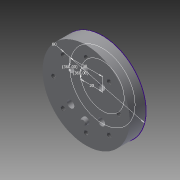
# Autodesk Inventor part: plate_for_CFS055CA501U
Saved by Autodesk Inventor 2013 (Build 170138000, 138)
## iProperties
Created: 2013-01-30
Part Number: plate_for_CFS055CA501U
Material: Generic
Document SubType Name: Modeling
Designer: Mahisorn
Density: 1 g/cm^3
Author: Mahisorn
Autodesk Inventor part; units mm, degrees
ref_plane "YZ Plane" through (0, 0, 0) normal (1, 0, 0) x (0, 1, 0)
ref_plane "XZ Plane" through (0, 0, 0) normal (0, 1, 0) x (-1, 0, 0)
ref_plane "XY Plane" through (0, 0, 0) normal (0, 0, 1) x (1, 0, 0)
sketch "Sketch1" plane through (0, 0, 0) normal (0, 1, 0) x (-1, 0, 0)
  circle A0 centre (0, 0) radius 40
  point P0 (20, 0)
  point P1 (14.1421, 14.1421)
  point P2 (0, 20)
  point P3 (-14.1421, 14.1421)
  point P4 (-20, 0)
  point P5 (-14.1421, -14.1421)
  point P6 (0, -20)
  point P7 (14.1421, -14.1421)
  point P8 (30, 0)
  point P9 (21.2132, 21.2132)
  point P10 (0, 30)
  point P11 (-21.2132, 21.2132)
  point P12 (-30, 0)
  point P13 (-21.2132, -21.2132)
  point P14 (0, -30)
  point P15 (21.2132, -21.2132)
  dimension "d0" = 80
  dimension "d2" = 20
  dimension "d5" = 360
  dimension "d31" = 30
  dimension "d34" = 360
  constraints: 5 coincident, 1 centre point, 30 other
  measures "d0" diameter of A0
  measures "d2" distance of point (20, 0) point (0, 0)
  measures "d31" distance of point (30, 0) point (0, 0)
extrude "Extrusion1" add sketch "Sketch1" against normal blind 15
hole "Hole1" at (-14.1421, 0, 14.1421) at (-14.1421, 0, -14.1421) at (14.1421, 0, 14.1421) at (14.1421, 0, -14.1421) direction (0, -1, 0) diameter 6.6 end through all counterbore diameter 11 counterbore depth 8 clearance for "Socket Head Cap Screw" size "M6" standard "Ansi Metric M Profile"
sketch "Sketch2" plane through (0, -15, 0) normal (0, -1, 0) x (1, 0, 0)
  circle A0 centre (0, 0) radius 40
  circle A1 centre (0, 20) radius 3
  circle A2 centre (0, -20) radius 3
  point P0 (20, 0)
  point P1 (14.1421, 14.1421)
  point P2 (-14.1421, 14.1421)
  point P3 (-20, 0)
  point P4 (-14.1421, -14.1421)
  point P5 (14.1421, -14.1421)
  dimension "d18" = 80
  dimension "d19" = 20
  dimension "d20" = 360
  dimension "d21" = 6
  dimension "d22" = 6
  constraints: 5 coincident, 3 centre point, 15 other
  measures "d18" diameter of A0
  measures "d19" distance of point (20, 0) point (0, 0)
  measures "d21" diameter of A1
  measures "d22" diameter of A2
extrude "Extrusion2" add sketch "Sketch2" along normal blind 3 contours A1 | A2
chamfer "Chamfer1" distance 1 angle 45 1 edges at (-3, -18, -20)
chamfer "Chamfer2" distance 1 angle 45 1 edges at (-3, -18, 20)
hole "Hole2" at (-30, 0, 0) at (-21.2132, 0, 21.2132) at (0, 0, 30) at (21.2132, 0, 21.2132) at (30, 0, 0) at (21.2132, 0, -21.2132) at (0, 0, -30) at (-21.2132, 0, -21.2132) direction (0, -1, 0) diameter 4.134 end through all thread size "M5x0.8" class "6H" standard "ANSI Metric M Profile"
body "Solid1"
